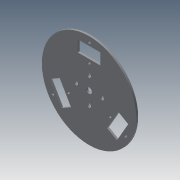
# Autodesk Inventor part: otocny_kruh
Saved by Autodesk Inventor 2013 (Build 170138000, 138)
## iProperties
Created: 2013-01-26
Part Number: otocny_kruh
Material: Generic
Document SubType Name: Modeling
Designer: idle-rug
Density: 1 g/cm^3
Author: idle-rug
Autodesk Inventor part; units mm, degrees
ref_plane "YZ Plane" through (0, 0, 0) normal (1, 0, 0) x (0, 1, 0)
ref_plane "XZ Plane" through (0, 0, 0) normal (0, 1, 0) x (-1, 0, 0)
ref_plane "XY Plane" through (0, 0, 0) normal (0, 0, 1) x (1, 0, 0)
sketch "Sketch1" plane through (0, 0, 0) normal (0, 1, 0) x (-1, 0, 0)
  circle A0 centre (0, 0) radius 50
  constraints: 1 centre point, 1 coincident
extrude "Extrusion1" add sketch "Sketch1" along normal blind 2
sketch "Sketch2" plane through (0, 0, 0) normal (0, -1, 0) x (1, 0, 0)
  circle A0 centre (0, 0) radius 50 projected
  circle A1 centre (0, 0) radius 3
  dimension "d3" = 6
  constraints: 1 centre point, 1 coincident
  measures "d3" diameter of A1
extrude "Extrusion2" cut sketch "Sketch2" against normal blind 2 contours A1
sketch "Sketch3" plane through (0, 0, 0) normal (0, -1, 0) x (1, 0, 0)
  circle A0 centre (0, 0) radius 50 projected
  circle A1 centre (0, 0) radius 11.5
  circle A2 centre (0, 0) radius 20
  circle A3 centre (0, 11.5) radius 2
  circle A4 centre (11.5, 0) radius 2
  circle A5 centre (-11.5, 0) radius 2
  circle A6 centre (0, -11.5) radius 2
  dimension "d15" = 23
  dimension "d16" = 40
  dimension "d17" = 4
  dimension "d18" = 4
  dimension "d19" = 4
  dimension "d20" = 4
  constraints: 6 centre point, 4 point on circle, 2 coincident
  measures "d15" diameter of A1
  measures "d16" diameter of A2
  measures "d17" diameter of A3
  measures "d18" diameter of A4
  measures "d19" diameter of A5
  measures "d20" diameter of A6
extrude "Extrusion3" cut sketch "Sketch3" against normal blind 2 contours A1 A4 | A1 A4 | A3 A1 | A1 A3 | A6 A1 | A1 A6 | A5 A1 | A1 A5
sketch "Sketch4" plane through (0, 0, 0) normal (0, -1, 0) x (1, 0, 0)
  circle A0 centre (0, -11.5) radius 2 projected
  circle A1 centre (11.5, 0) radius 2 projected
  circle A2 centre (0, 11.5) radius 2 projected
  circle A3 centre (-11.5, 0) radius 2 projected
extrude "Extrusion4" add sketch "Sketch4" against normal blind 2
sketch "Sketch5" plane through (0, 2, 0) normal (0, 1, 0) x (1, 0, 0)
  circle A0 centre (0, 0) radius 50 projected
  circle A1 centre (0, 0) radius 13.75
  circle A2 centre (0, 13.75) radius 2
  circle A3 centre (13.75, 0) radius 2
  circle A4 centre (0, -13.75) radius 2
  circle A5 centre (-13.75, 0) radius 2
  dimension "d25" = 27.5
  dimension "d26" = 4
  dimension "d27" = 4
  dimension "d28" = 4
  dimension "d29" = 4
  constraints: 5 centre point, 4 point on circle, 1 coincident
  measures "d25" diameter of A1
  measures "d26" diameter of A2
  measures "d27" diameter of A3
  measures "d28" diameter of A4
  measures "d29" diameter of A5
extrude "Extrusion5" cut sketch "Sketch5" against normal blind 2 contours A1 A3 | A1 A3 | A2 A1 | A1 A2 | A4 A1 | A1 A4 | A5 A1 | A1 A5
sketch "Sketch6" plane through (0, 0, 0) normal (0, -1, 0) x (1, 0, 0)
  circle A0 centre (0, 0) radius 50 projected
  line L0 (0, 0) -> (0, 50)
  line L1 (0, 0) -> (50, 0) construction
  line L2 (0, 0) -> (50, 0) construction
  line L3 (-12, 40) -> (12, 40)
  line L4 (12, 40) -> (12, 30)
  line L5 (12, 30) -> (-12, 30)
  line L6 (-12, 30) -> (-12, 40)
  line L7 (-12, 40) -> (12, 30) construction
  line L8 (12, 40) -> (-12, 30) construction
  line L9 (-30.3109, -17.5) -> (-25.9808, -15)
  line L10 (-25.9808, -15) -> (-34.641, -20)
  line L11 (-34.641, -20) -> (-28.641, -30.3923)
  line L12 (-28.641, -30.3923) -> (-19.641, -25.1962)
  line L13 (-19.641, -25.1962) -> (-31.641, -4.4115)
  line L14 (-28.641, -30.3923) -> (-40.641, -9.6077)
  line L15 (-40.641, -9.6077) -> (-31.641, -4.4115)
  line L16 (25.9808, -15) -> (19.9808, -25.3923)
  line L17 (19.9808, -25.3923) -> (28.641, -30.3923)
  line L18 (28.641, -30.3923) -> (40.641, -9.6077)
  line L19 (40.641, -9.6077) -> (31.9808, -4.6077)
  line L20 (31.9808, -4.6077) -> (25.9808, -15)
  point P0 (0, 35)
  dimension "d35" = 24
  dimension "d36" = 10
  dimension "d38" = 10
  dimension "d39" = 12
  dimension "d41" = 24
  dimension "d44" = 12
  dimension "d45" = 10
  dimension "d46" = 24
  dimension "d47" = 10
  constraints: 42 end point, 5 perpendicular, 3 horizontal, 3 parallel, 2 midpoint, 1 point on line, 1 vertical, 1 vertical alignment, 1 other
  measures "d35" distance of L4.end L5.end
  measures "d36" distance of L3.end L4.end
  measures "d38" distance of L9.end L10.end
  measures "d39" distance of L10.end L11.end
  measures "d41" distance of L11.end L14.end
  measures "d44" distance of L16.start L16.end
  measures "d45" distance of L16.end L17.end
  measures "d46" distance of L17.end L18.end
  measures "d47" distance of L18.end L19.end
extrude "Extrusion6" cut sketch "Sketch6" against normal blind 2 contours L5 L6 L3 L0 | L0 L3 L4 L5 | L14 L15 L13 L12 L11 | L20 L19 L18 L17 L16
sketch "Sketch7" plane through (0, 0, 0) normal (0, -1, 0) x (1, 0, 0)
  line L0 (28.641, -30.3923) -> (19.9808, -25.3923) projected
  line L1 (31.9808, -4.6077) -> (40.641, -9.6077) projected
  line L2 (40.641, -9.6077) -> (28.641, -30.3923) projected
  line L3 (-12, 30) -> (-12, 40) projected
  line L4 (-12, 40) -> (12, 40) projected
  line L5 (12, 40) -> (12, 30) projected
  line L6 (12, 30) -> (-12, 30) projected
  line L7 (-31.641, -4.4115) -> (-19.641, -25.1962) projected
  line L8 (-19.641, -25.1962) -> (-28.641, -30.3923) projected
  line L9 (-28.641, -30.3923) -> (-40.641, -9.6077) projected
  line L10 (-40.641, -9.6077) -> (-31.641, -4.4115) projected
  line L11 (12, 42) -> (-12, 42)
  line L12 (-12, 42) -> (-12, 28)
  line L13 (-12, 28) -> (12, 28)
  line L14 (12, 28) -> (12, 42)
  line L15 (12, 42) -> (-12, 28) construction
  line L16 (-12, 42) -> (12, 28) construction
  line L17 (-36.141, -7.0096) -> (-30.0788, -3.5096)
  line L18 (-30.0788, -3.5096) -> (-18.0788, -24.2942)
  line L19 (-18.0788, -24.2942) -> (-30.2032, -31.2942)
  line L20 (-30.2032, -31.2942) -> (-42.2032, -10.5096)
  line L21 (-42.2032, -10.5096) -> (-36.141, -7.0096)
  line L22 (36.3109, -7.1077) -> (30.2644, -3.5806)
  line L23 (30.2644, -3.5806) -> (18.1715, -24.3113)
  line L24 (18.1715, -24.3113) -> (30.2801, -31.3386)
  line L25 (30.2801, -31.3386) -> (42.2801, -10.554)
  line L26 (42.2801, -10.554) -> (30.2644, -3.5806)
  point P0 (0, 35)
  dimension "d50" = 24
  dimension "d51" = 14
  dimension "d52" = 7
  dimension "d53" = 24
  dimension "d54" = 14
  dimension "d55" = 24
  dimension "d56" = 7
  dimension "d57" = 24
  dimension "d58" = 14
  dimension "d59" = 24
  constraints: 32 end point, 5 parallel, 4 midpoint, 3 perpendicular, 3 point on line, 1 horizontal
  measures "d50" distance of L13.end L12.end
  measures "d51" distance of L12.end L11.end
  measures "d52" distance of L17.start L17.end
  measures "d53" distance of L17.end L18.end
  measures "d54" distance of L18.end L19.end
  measures "d55" distance of L19.end L20.end
  measures "d56" distance of L22.start L22.end
  measures "d57" distance of L22.end L23.end
  measures "d58" distance of L23.end L24.end
  measures "d59" distance of L24.end L25.end
extrude "Extrusion7" cut sketch "Sketch7" against normal blind 2 contours L22 L26 L25 L24 L2 L1 | L1 L2 L24 L23 L22 | L6 L14 L13 L12 | L12 L11 L14 L4 | L17 L18 L19 L7 | L19 L20 L21 L9
sketch "Sketch8" plane through (0, 0, 0) normal (0, -1, 0) x (1, 0, 0)
  line L0 (30.2801, -31.3386) -> (28.6432, -30.3886) projected
  line L1 (28.641, -30.3923) -> (19.9808, -25.3923) projected
  line L2 (19.9942, -25.3691) -> (18.1715, -24.3113) projected
  line L3 (18.1715, -24.3113) -> (30.2644, -3.5806) projected
  line L4 (30.2644, -3.5806) -> (42.2801, -10.554) projected
  line L5 (42.2801, -10.554) -> (30.2801, -31.3386) projected
  line L6 (-42.2032, -10.5096) -> (-30.0788, -3.5096) projected
  line L7 (-30.0788, -3.5096) -> (-18.0788, -24.2942) projected
  line L8 (-18.0788, -24.2942) -> (-30.2032, -31.2942) projected
  line L9 (-30.2032, -31.2942) -> (-42.2032, -10.5096) projected
  line L10 (-12, 28) -> (-12, 42) projected
  line L11 (-12, 42) -> (12, 42) projected
  line L12 (12, 42) -> (12, 28) projected
  line L13 (12, 28) -> (-12, 28) projected
  line L14 (12, 41) -> (-12, 41)
  line L15 (-12, 41) -> (-12, 29)
  line L16 (-12, 29) -> (12, 29)
  line L17 (12, 29) -> (12, 41)
  line L18 (12, 41) -> (-12, 29) construction
  line L19 (-12, 41) -> (12, 29) construction
  line L20 (-36.141, -7.0096) -> (-30.9449, -4.0096)
  line L21 (-30.9449, -4.0096) -> (-18.9449, -24.7942)
  line L22 (-18.9449, -24.7942) -> (-29.3372, -30.7942)
  line L23 (-29.3372, -30.7942) -> (-41.3372, -10.0096)
  line L24 (-41.3372, -10.0096) -> (-36.141, -7.0096)
  line L25 (24.3109, -27.8923) -> (29.508, -30.8906)
  line L26 (29.508, -30.8906) -> (41.5081, -10.106)
  line L27 (41.5081, -10.106) -> (31.1293, -4.0826)
  line L28 (31.1293, -4.0826) -> (19.0829, -24.8402)
  line L29 (19.0829, -24.8402) -> (24.3109, -27.8923)
  point P0 (0, 35)
  dimension "d62" = 24
  dimension "d63" = 12
  dimension "d64" = 6
  dimension "d65" = 24
  dimension "d66" = 12
  dimension "d67" = 24
  dimension "d68" = 6
  dimension "d69" = 24
  dimension "d70" = 12
  constraints: 32 end point, 7 point on line, 5 midpoint, 2 parallel, 1 collinear, 1 horizontal, 1 perpendicular
  measures "d62" distance of L16.end L15.end
  measures "d63" distance of L15.end L14.end
  measures "d64" distance of L20.start L20.end
  measures "d65" distance of L20.end L21.end
  measures "d66" distance of L21.end L22.end
  measures "d67" distance of L22.end L23.end
  measures "d68" distance of L25.start L25.end
  measures "d69" distance of L25.end L26.end
  measures "d70" distance of L26.end L27.end
extrude "Extrusion8" add sketch "Sketch8" against normal blind 2 contours L0 L26 L4 L5 | L28 L2 L3 L4 | L6 L23 L8 L9 | L6 L7 L8 L21 | L10 L16 L12 L13 | L10 L11 L12 L14
sketch "Sketch11" plane through (0, 0, 0) normal (0, -1, 0) x (1, 0, 0)
  line L0 (29.508, -30.8906) -> (28.6432, -30.3886) projected
  line L1 (28.6432, -30.3886) -> (28.641, -30.3923) projected
  line L2 (28.641, -30.3923) -> (19.9808, -25.3923) projected
  line L3 (19.9808, -25.3923) -> (19.9942, -25.3691) projected
  line L4 (19.9942, -25.3691) -> (19.0829, -24.8402) projected
  line L5 (19.0829, -24.8402) -> (31.1293, -4.0826) projected
  line L6 (31.1293, -4.0826) -> (41.5081, -10.106) projected
  line L7 (41.5081, -10.106) -> (29.508, -30.8906) projected
  line L8 (-41.3372, -10.0096) -> (-30.9449, -4.0096) projected
  line L9 (-30.9449, -4.0096) -> (-18.9449, -24.7942) projected
  line L10 (-18.9449, -24.7942) -> (-29.3372, -30.7942) projected
  line L11 (-29.3372, -30.7942) -> (-41.3372, -10.0096) projected
extrude "Extrusion9" add sketch "Sketch11" against normal blind 2
sketch "Sketch12" plane through (0, 0, 0) normal (0, -1, 0) x (1, 0, 0)
  line L0 (-12, 41) -> (12, 41) projected
  line L1 (12, 29) -> (-12, 29) projected
  circle A0 centre (0, 0) radius 50 projected
  line L2 (0, 0) -> (35, 0) construction
  line L3 (0, 0) -> (35, 0) construction
  line L4 (0, 41) -> (0, 29)
  line L5 (25.1147, -14.5) -> (19.1147, -24.8923)
  line L6 (19.1147, -24.8923) -> (29.507, -30.8923)
  line L7 (29.507, -30.8923) -> (41.507, -10.1077)
  line L8 (41.507, -10.1077) -> (31.1147, -4.1077)
  line L9 (31.1147, -4.1077) -> (25.1147, -14.5)
  line L10 (-25.1147, -14.5) -> (-31.1147, -4.1077)
  line L11 (-31.1147, -4.1077) -> (-41.507, -10.1077)
  line L12 (-41.507, -10.1077) -> (-29.507, -30.8923)
  line L13 (-29.507, -30.8923) -> (-19.1147, -24.8923)
  line L14 (-19.1147, -24.8923) -> (-25.1147, -14.5)
  line L15 (19.1147, -24.8923) -> (31.1147, -4.1077)
  line L16 (31.1147, -4.1077) -> (41.507, -10.1077)
  line L17 (41.507, -10.1077) -> (29.507, -30.8923)
  line L18 (29.507, -30.8923) -> (19.1147, -24.8923)
  line L19 (-41.507, -10.1077) -> (-31.1147, -4.1077)
  line L20 (-31.1147, -4.1077) -> (-19.1147, -24.8923)
  line L21 (-19.1147, -24.8923) -> (-29.507, -30.8923)
  line L22 (-29.507, -30.8923) -> (-41.507, -10.1077)
  dimension "d92" = 12
  dimension "d93" = 12
  dimension "d94" = 12
  dimension "d97" = 12
  constraints: 42 end point, 8 perpendicular, 4 parallel, 2 horizontal, 2 midpoint, 1 coincident
  measures "d92" distance of L5.start L5.end
  measures "d93" distance of L7.end L8.end
  measures "d94" distance of L8.end L5.start
  measures "d97" distance of L13.start L13.end
extrude "Extrusion10" cut sketch "Sketch12" against normal blind 2 contours L9 L8 L7 L6 L5 | L14 L13 L12 L11 L10
sketch "Sketch14" plane through (0, 0, 0) normal (0, -1, 0) x (1, 0, 0)
  line L0 (12, 29) -> (-12, 29) projected
  circle A0 centre (-38.5381, -22.25) radius 1.5
  circle A1 centre (-22.0836, -12.75) radius 1.5
  circle A2 centre (0, 44.5) radius 1.5
  line L1 (0, 41) -> (0, 29)
  circle A3 centre (0, 25.5) radius 1.5
  circle A4 centre (38.5381, -22.25) radius 1.5
  circle A5 centre (22.0836, -12.75) radius 1.5
  dimension "d107" = 3
  dimension "d108" = 3
  dimension "d109" = 3
  dimension "d110" = 3
  dimension "d112" = 3
  constraints: 6 centre point, 2 end point, 1 midpoint
  measures "d107" diameter of A0
  measures "d108" diameter of A1
  measures "d109" diameter of A2
  measures "d110" diameter of A3
  measures "d112" diameter of A5
extrude "Extrusion11" cut sketch "Sketch14" against normal blind 2
body "Solid1"
